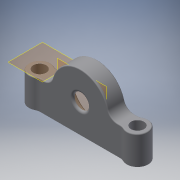
# Autodesk Inventor part: Pillow Block
Saved by Autodesk Inventor 2016 (Build 200138000, 138)
## iProperties
Created: 2016-02-11
Part Number: Pillow Block
Material: Generic
Document SubType Name: Modeling
Designer: Spooner
Density: 1 g/cm^3
Appearance: Default
Author: Spooner
Autodesk Inventor part; units mm, degrees
ref_plane "YZ Plane" through (0, 0, 0) normal (1, 0, 0) x (0, 1, 0)
ref_plane "Work Plane1" through (0, 0, 0) normal (0, 0, 1) x (1, 0, 0)
sketch "Sketch1" plane through (0, 0, 0) normal (0, 0, 1) x (1, 0, 0)
  circle A0 centre (0, 0) radius 4.7625 projected
  circle A1 centre (0, 0) radius 14.2875 projected
  circle A2 centre (0, 0) radius 14.351
  circle A3 centre (0, 0) radius 20.701
  line L0 (-20.701, 0) -> (-39.751, 0)
  line L1 (-39.751, 0) -> (-39.751, -20.701)
  line L2 (-39.751, -20.701) -> (39.751, -20.701)
  line L3 (39.751, -20.701) -> (39.751, 0)
  line L4 (39.751, 0) -> (20.701, 0)
  point P0 (0, 0)
  dimension "d0" = 0.0635
  dimension "d1" = 6.35
  dimension "d2" = 19.05
  constraints: 10 end point, 3 perpendicular, 2 centre point, 2 coincident, 2 point on circle, 2 point on line, 1 collinear, 1 horizontal, 1 horizontal alignment, 1 tangent
  measures "d0" radial gap between concentric circles of A1 A2
  measures "d1" radial gap between concentric circles of A3 A2
  measures "d2" distance of L0.start L0.end
ref_plane "Work Plane2" through (-14.2875, -14.2875, -9.525) normal (0, 0, -1) x (0, 1, 0)
ref_plane "Work Plane4" through (-14.2875, -14.2875, -19.05) normal (0, 0, -1) x (0, 1, 0)
extrude "Extrusion1" add sketch "Sketch1" against normal up to surface (19.05 mm away) contours A3 | L4 L3 L2 A3 | A3 L2 L1 L0
fillet "Fillet1" radius 6.35 2 edges at (-20.701, 0, -9.525) (20.701, 0, -9.525)
sketch "Sketch2" plane through (0, 0, 0) normal (0, 0, 1) x (1, 0, 0)
  circle A0 centre (0, 0) radius 14.351 projected
  line L0 (-26.2951, 0) -> (-39.751, 0) projected
  line L1 (-39.751, 0) -> (-39.751, -20.701) projected
  line L2 (-39.751, -20.701) -> (39.751, -20.701) projected
  line L3 (39.751, -20.701) -> (39.751, 0) projected
  line L4 (39.751, 0) -> (26.2951, 0) projected
  arc A1 (20.1226, 4.8594) -> (26.2951, 0) centre (26.2951, 6.35) ccw projected
  arc A2 (20.1226, 4.8594) -> (-20.1226, 4.8594) centre (0, 0) ccw projected
  arc A3 (-26.2951, 0) -> (-20.1226, 4.8594) centre (-26.2951, 6.35) ccw projected
  circle A4 centre (0, 0) radius 4.7625 projected
  circle A5 centre (0, 0) radius 6.0325
  point P0 (0, 0)
  dimension "d6" = 1.27
  constraints: 1 centre point, 1 coincident
  measures "d6" radial gap between concentric circles of A4 A5
extrude "Extrusion2" add sketch "Sketch2" along normal blind 1.27 contours A0 | A3 A2 A1 L4 L3 L2 L1 L0 | A5
fillet "Fillet2" radius 3.175 4 edges at (-39.751, -10.3505, 1.27) (-39.751, -10.3505, -19.05) (39.751, -10.3505, 1.27) (39.751, -10.3505, -19.05)
fillet "Fillet4" radius 1.5875 1 edges at (-4.7625, 0, 1.27)
chamfer "Chamfer1" distance 1.27 angle 45 1 edges at (-14.351, 0, -19.05)
ref_plane "Work Plane3" through (-34.036, 0, -8.763) normal (0, 1, 0) x (1, 0, 0)
sketch "Sketch3" plane through (-34.036, 0, -8.763) normal (0, 1, 0) x (1, 0, 0)
  line L0 (60.3311, -10.033) -> (60.3311, 10.287) projected
  line L1 (7.7409, 10.287) -> (7.7409, -10.033) projected
  circle A0 centre (66.6115, 0.127) radius 4.1275
  circle A1 centre (-121.701, -3.81) radius 4.1275
  circle A2 centre (1.4605, 0.127) radius 4.1275
  arc A3 (-2.54, 10.287) -> (-5.715, 7.112) centre (-2.54, 7.112) ccw projected
  line L2 (-5.715, 7.112) -> (-5.715, -6.858) projected
  arc A4 (-5.715, -6.858) -> (-2.54, -10.033) centre (-2.54, -6.858) ccw projected
  line L3 (7.7409, -10.033) -> (-2.54, -10.033) projected
  line L4 (7.7409, 10.287) -> (-2.54, 10.287) projected
  arc A5 (73.787, 7.112) -> (70.612, 10.287) centre (70.612, 7.112) ccw projected
  line L5 (70.612, 10.287) -> (60.3311, 10.287) projected
  line L6 (70.612, -10.033) -> (60.3311, -10.033) projected
  arc A6 (70.612, -10.033) -> (73.787, -6.858) centre (70.612, -6.858) ccw projected
  line L7 (73.787, 7.112) -> (73.787, -6.858) projected
  point P0 (34.036, -8.763)
  point P1 (71.247, 0.127)
  point P2 (73.787, 0.127)
  dimension "d15" = 8.255
  dimension "d20" = 3.048
  dimension "d21" = 3.048
  constraints: 3 centre point, 3 horizontal alignment, 2 equal radius, 1 midpoint
  measures "d15" diameter of A0
  measures "d20" distance edge to line of A2 L2
  measures "d21" distance edge to line of A0 L7
extrude "Extrusion3" cut sketch "Sketch3" against normal through all contours A0 | A2
fillet "Fillet6" radius 0.635 10 edges at (31.4356, 0, 1.27) (22.3672, 1.3606, 1.27) (0, 20.701, 1.27) (-22.3672, 1.3606, 1.27) (-31.4356, 0, 1.27) (-31.4356, 0, -19.05) (31.4356, 0, -19.05) (-22.3672, 1.3606, -19.05) (0, 20.701, -19.05) (22.3672, 1.3606, -19.05)
equation "\"d21\" = d20"
body "Solid1"
